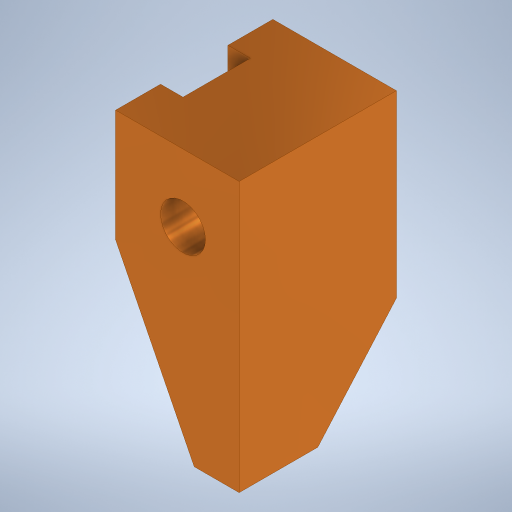
# Autodesk Inventor part: ASN5-3-BK
Saved by Autodesk Inventor 2024 (Build 280153000, 153)
## iProperties
Created: 2023-10-06
Part Number: ASN5-3-BK
Material: Gold
Document SubType Name: Modeling
Designer: bennk
Density: 19.3 g/cm^3
Appearance: Metal 1600F Hot
Mass: 12555.6 g
Surface Area: 583.698 cm^2
Volume: 650.55 cm^3
Author: bennk
Autodesk Inventor part; units mm, degrees
ref_plane "YZ Plane" through (0, 0, 0) normal (1, 0, 0) x (0, 1, 0)
ref_plane "XZ Plane" through (0, 0, 0) normal (0, 1, 0) x (-1, 0, 0)
ref_plane "XY Plane" through (0, 0, 0) normal (0, 0, 1) x (1, 0, 0)
sketch "Sketch1" plane through (0, 0, 0) normal (0, 1, 0) x (-1, 0, 0)
  line L0 (69.85, 44.45) -> (0, 44.45)
  line L1 (0, 44.45) -> (0, -44.45)
  line L2 (0, -44.45) -> (69.85, -44.45)
  line L3 (69.85, -44.45) -> (69.85, 44.45)
  line L4 (69.85, 19.05) -> (57.15, 19.05)
  line L5 (57.15, 19.05) -> (57.15, -19.05)
  line L6 (57.15, -19.05) -> (69.85, -19.05)
  line L7 (69.85, -19.05) -> (69.85, 19.05)
  point P0 (0, 0)
  point P1 (0, 0)
  dimension "d0" = 88.9
  dimension "d1" = 69.85
  dimension "d3" = 12.7
  dimension "d4" = 38.1
  dimension "d5" = 19.05
  dimension "d6" = 0
  dimension "d7" = 44.45
  constraints: 16 end point, 4 parallel, 2 horizontal, 2 midpoint, 2 perpendicular
  measures "d0" distance of L0.end L1.end
  measures "d1" distance of L0.start L0.end
  measures "d3" distance between parallel lines of L7 L5
  measures "d4" distance of L6.end L4.start
  measures "d5" distance from line of point (0, 0) L4
  measures "d6" distance between parallel lines of L3 L7
  measures "d7" distance from line of point (0, 0) L2
extrude "NOTCHED SHAPE" add sketch "Sketch1" along normal blind 152.4 contours L3 L4 L5 L6 L2 L1 L0
chamfer "TOP SURF" distance 88.9 distance2 44.45 1 edges at (-69.85, 0, 31.75) measured on face at (-69.85, 0.5, 31.75)
chamfer "EDGE SURF" distance 44.45 distance2 50.8 1 edges at (-12.7, 0, -44.45) measured on face at (-12.7, 0, -43.95)
sketch "Sketch2" plane through (0, 152.4, -44.45) normal (0, 0, -1) x (-1, 0, 0)
  line L0 (0, 0) -> (69.85, 0) projected
  line L1 (0, -101.6) -> (0, 0) projected
  point P0 (0, -152.4)
  point P1 (31.75, -38.1)
  dimension "d16" = 38.1
  dimension "d17" = 31.75
  measures "d16" distance from line of L0 point (31.75, -38.1)
  measures "d17" distance from line of L1 point (31.75, -38.1)
hole "Hole1" at (-31.75, 114.3, -44.45) direction (0, 0, 1) diameter 25.4 end through all
equation "\"d5\" = 0.5 * d4"
equation "\"d7\" = 0.5 * d0"
body "Solid1"
